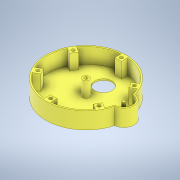
# Autodesk Inventor part: filterBase
Saved by Autodesk Inventor 2022.1 (Build 261234020, 234B)
## iProperties
Created: 2020-04-12
Part Number: filterBase
Material: PBT Plastic
Document SubType Name: Modeling
Designer: robst
Density: 1.31 g/cm^3
Appearance: Smooth - Yellow
Author: robst
Autodesk Inventor part; units mm, degrees
ref_plane "YZ Plane" through (0, 0, 0) normal (1, 0, 0) x (0, 1, 0)
ref_plane "XZ Plane" through (0, 0, 0) normal (0, 1, 0) x (-1, 0, 0)
ref_plane "XY Plane" through (0, 0, 0) normal (0, 0, 1) x (1, 0, 0)
sketch "Sketch3" plane through (0, 0, 0) normal (0, 0, 1) x (1, 0, 0)
  line L0 (0, 0) -> (76.2, 0)
  line L1 (76.2, 0) -> (76.2, 31.75)
  line L2 (76.2, 31.75) -> (73.66, 31.75)
  line L3 (73.66, 31.75) -> (73.66, 2.54)
  line L4 (73.66, 2.54) -> (0, 2.54)
  line L5 (0, 2.54) -> (0, 0)
  dimension "d3" = 76.2
  dimension "d4" = 31.75
  dimension "d5" = 2.54
  dimension "d15" = 2.54
  constraints: 12 end point, 3 perpendicular, 2 horizontal, 1 parallel
  measures "d3" distance of L0.start L0.end
  measures "d4" distance of L0.end L1.end
  measures "d5" distance of L1.end L2.end
  measures "d15" distance between parallel lines of L4 L0
revolve "Revolution1" add sketch "Sketch3" angle 360 about axis through (0, 2.54, 0) along (0, -1, 0)
sketch "Sketch4" plane through (0, 2.54, 0) normal (0, 1, 0) x (1, 0, 0)
  circle A0 centre (0, 0) radius 6.223
  point P0 (0, 0)
  dimension "d8" = 12.446
  constraints: 1 centre point, 1 coincident
  measures "d8" diameter of A0
extrude "Extrusion2" add sketch "Sketch4" along normal blind 29.21
sketch "Sketch5" plane through (0, 2.54, 0) normal (0, 1, 0) x (1, 0, 0)
  circle A0 centre (0, 33.165605) radius 16.256
  point P0 (0, 0)
  dimension "d11" = 33.16561
  dimension "d12" = 32.512
  constraints: 1 centre point
  measures "d11" distance of A0.centre point (0, 0)
  measures "d12" diameter of A0
extrude "HoleForTelescopeInsert" cut sketch "Sketch5" against normal through all
sketch "Sketch6" plane through (0, 31.75, 0) normal (0, 1, 0) x (1, 0, 0)
  circle A0 centre (0, 0) radius 6.223 projected
  point P0 (0, 0)
  point P1 (0, 0)
  constraints: 1 coincident
hole "Hole1" at (0, 31.75, 0) direction (0, -1, 0) diameter 6.3246 depth 14.605 counterbore diameter 6.5278 counterbore depth 7.62
sketch "Sketch8" plane through (0, 2.54, 0) normal (0, 1, 0) x (1, 0, 0)
  circle A0 centre (0, 0) radius 3.1623
  arc A1 (-6.35, -61.266806) -> (6.35, -61.266806) centre (0, 0) ccw
  circle A2 centre (0, 0) radius 73.66
  line L0 (-6.35, -73.385783) -> (-6.35, -61.266806)
  line L1 (6.35, -73.385783) -> (6.35, -61.266806)
  point P0 (0, 0)
  dimension "d27" = 123.19
  dimension "d28" = 12.7
  constraints: 4 end point, 4 point on circle, 2 vertical, 1 centre point, 1 coincident, 1 parallel
  measures "d27" diameter of A1
  measures "d28" distance between parallel lines of L0 L1
extrude "Extrusion5" add sketch "Sketch8" along normal blind 29.21 contours A1 L1 A2 L0 picked at (4.940005, -65.403698)
sketch "Sketch10" plane through (0, 31.75, 0) normal (0, 1, 0) x (1, 0, 0)
  line L0 (-6.35, -73.385783) -> (-6.35, -61.266806) construction
  arc A0 (-6.35, -61.266806) -> (6.35, -61.266806) centre (0, 0) ccw construction
  line L1 (-6.35, -73.385783) -> (6.35, -61.266806) construction
  line L2 (6.35, -61.266806) -> (-6.35, -61.266806) construction
  line L3 (6.35, -61.266806) -> (6.35, -73.385783) construction
  line L4 (6.35, -73.385783) -> (-6.35, -61.266806) construction
  point P0 (0, 0)
  point P1 (0, -67.326294)
  constraints: 6 end point, 1 horizontal, 1 midpoint
hole "Hole4" at (0, 31.75, 67.326294) direction (0, -1, 0) diameter 5.5372 depth 9.525 counterbore diameter 6.3246 counterbore depth 6.15188
pattern_circular "Circular Pattern1" count 6 over 360 about axis through (0, -10, 0) along (0, 1, 0) of "Extrusion5", "Hole4"
sketch "Sketch12" plane through (0, 31.75, 0) normal (0, 1, 0) x (1, 0, 0)
  circle A0 centre (0, 0) radius 3.2639 construction
  arc A1 (74.125667, -17.658583) -> (74.125667, 17.658583) centre (0, 0) ccw
  line L0 (0, 0) -> (76.2, 0) construction
  circle A2 centre (0, 0) radius 76.2 construction
  line L1 (0, 0) -> (74.125667, 17.658583) construction
  line L2 (0, 0) -> (74.125667, -17.658583) construction
  arc A3 (71.654811, -17.069963) -> (71.654811, 17.069963) centre (0, 0) ccw
  line L3 (71.654811, 17.069963) -> (74.125667, 17.658583) construction
  line L4 (71.654811, 17.069963) -> (74.125667, 17.658583)
  line L5 (71.654811, -17.069963) -> (74.125667, -17.658583)
  point P0 (0, 0)
  dimension "d55" = 17.78
  dimension "d56" = 13.3995
  dimension "d58" = 17.78
  constraints: 12 end point, 7 point on circle, 3 collinear, 2 centre point, 2 coincident, 2 point on line, 1 horizontal
  measures "d55" distance of L1.end L0.end
  measures "d56" angle of L1 L0
  measures "d58" distance of L0.end L2.end
extrude "Extrusion6" cut sketch "Sketch12" against normal blind 29.21
sketch "Sketch13" plane through (0, 0, 0) normal (0, -1, 0) x (1, 0, 0)
  circle A0 centre (0, 0) radius 3.1623 construction
  line L0 (0, 0) -> (76.2, 0) construction
  arc A1 (74.125667, -17.658583) -> (74.125667, 17.658583) centre (0, 0) ccw construction
  circle A2 centre (71.755, 0) radius 3.048
  point P0 (0, 0)
  dimension "d61" = 6.096
  dimension "d62" = 71.755
  constraints: 2 end point, 1 centre point, 1 horizontal, 1 point on circle, 1 point on line
  measures "d61" diameter of A2
  measures "d62" distance of A2.centre point (0, 0)
extrude "Extrusion7" add sketch "Sketch13" against normal blind 29.21
sketch "Sketch14" plane through (0, 0, 0) normal (0, -1, 0) x (1, 0, 0)
  circle A0 centre (71.755, 0) radius 3.048
  arc A1 (74.3072, -16.878387) -> (74.3072, 16.878387) centre (71.755, 0) ccw
  arc A2 (73.657988, -19.517705) -> (73.657988, 19.517705) centre (71.755, 0) ccw
  arc A3 (73.657988, -19.517705) -> (74.3072, -16.878387) centre (0, 0) ccw
  arc A4 (74.3072, 16.878387) -> (73.657988, 19.517705) centre (0, 0) ccw
  point P0 (0, 0)
  point P1 (71.654811, 17.069963)
  point P2 (71.654811, -17.069963)
  dimension "d65" = 2.54
  constraints: 9 point on circle, 4 centre point, 2 coincident
  measures "d65" radial gap between concentric circles of A1 A2
extrude "Extrusion8" add sketch "Sketch14" against normal blind 31.75 contours A1 A4 A2 A3
sketch "Sketch15" plane through (0, 31.75, 0) normal (0, 1, 0) x (1, 0, 0)
  line L0 (74.125667, -17.658583) -> (71.654811, -17.069963)
  arc A0 (74.3072, -16.878387) -> (74.3072, 16.878387) centre (0, 0) ccw
  arc A1 (74.125667, -17.658583) -> (74.3072, -16.878387) centre (0, 0) ccw
  arc A2 (74.3072, 16.878387) -> (74.125667, 17.658583) centre (0, 0) ccw
  line L1 (71.654811, 17.069963) -> (74.125667, 17.658583)
  arc A3 (74.3072, -16.878387) -> (74.3072, 16.878387) centre (71.755, 0) ccw
  arc A4 (73.657988, -19.517705) -> (73.657988, 19.517705) centre (71.755, 0) ccw
  arc A5 (6.35, -73.385783) -> (71.654811, -17.069963) centre (0, 0) ccw
  line L2 (74.125667, -17.658583) -> (71.654811, -17.069963)
  line L3 (71.654811, -17.069963) -> (74.125667, -17.658583)
  line L4 (74.125667, -17.658583) -> (74.3072, -16.878387)
  arc A6 (71.654811, 17.069963) -> (60.378952, -42.192153) centre (0, 0) ccw
  line L5 (71.654811, 17.069963) -> (74.125667, 17.658583)
  arc A7 (74.3072, 16.878387) -> (74.125667, 17.658583) centre (0, 0) ccw
  line L6 (74.125667, 17.658583) -> (74.3072, 16.878387)
  arc A8 (71.654811, -17.069963) -> (74.3072, -16.878387) centre (71.755, 0) ccw
  arc A9 (74.3072, 16.878387) -> (71.654811, 17.069963) centre (71.755, 0) ccw
  constraints: 8 end point, 6 point on circle, 2 centre point, 1 coincident, 1 collinear
sketch "Sketch15 outline for Extrusion9" plane through (0, 31.75, 0) normal (0, 1, 0) x (1, 0, 0)
  arc A0 (71.654811, 17.069963) -> (74.3072, 16.878387) centre (71.755, 0) cw
  line L0 (74.125667, 17.658583) -> (71.654811, 17.069963)
  line L1 (74.3072, 16.878387) -> (74.125667, 17.658583)
  line L2 (74.125667, -17.658583) -> (74.3072, -16.878387)
  line L3 (71.654811, -17.069963) -> (74.125667, -17.658583)
  arc A1 (74.3072, -16.878387) -> (71.654811, -17.069963) centre (71.755, 0) cw
extrude "Extrusion9" add sketch "Sketch15 outline for Extrusion9" against normal up to surface (29.21 mm away)
sketch "Sketch16" plane through (71.755, 0, 0) normal (0, -1, 0) x (1, 0, 0)
  arc A0 (2.5522, -16.878387) -> (2.5522, 16.878387) centre (0, 0) ccw
  arc A1 (2.5522, -16.878387) -> (2.5522, 16.878387) centre (-71.755, 0) ccw
  circle A2 centre (0, 0) radius 3.048
  arc A3 (2.5522, -16.878387) -> (2.5522, 16.878387) centre (0, 0) ccw
  circle A4 centre (-71.755, 0) radius 3.1623
  arc A5 (2.5522, -16.878387) -> (2.5522, 16.878387) centre (-71.755, 0) ccw
  constraints: 4 point on circle, 2 centre point, 2 coincident
extrude "Extrusion10" add sketch "Sketch16" against normal up to surface (2.54 mm away) contours A1 A0
equation "\"d4\" = height"
equation "\"d8\" = centerHoleDiameter"
equation "\"d9\" = postHeight"
equation "\"height\" = 31.75"
equation "\"outerDiameter\" = 129.54"
equation "\"outerRadius\" = 0.5 * outerDiameter"
equation "\"centerHoleDiameter\" = 12.446"
equation "\"postHeight\" = height - baseThickness"
equation "\"baseThickness\" = 2.54"
body "Solid2"
